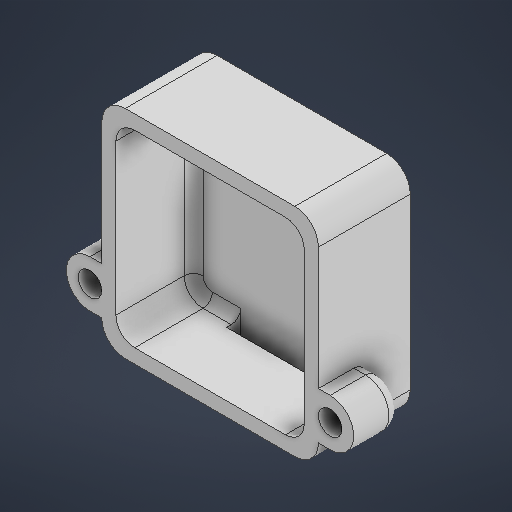
# Autodesk Inventor part: FANHOLDER
Saved by Autodesk Inventor 2025 (Build 290162010, 162A)
## iProperties
Created: 2024-04-29
Part Number: FANHOLDER
Material: Generic
Document SubType Name: Modeling
Designer: techn
Density: 1 g/cm^3
Appearance: Default
Author: techn
## iProperties of the stored document FANHOLDER_3DPrint.ipt
Created: 2024-05-28
Part Number: FANHOLDER_3DPrint
Material: Generic
Document SubType Name: Modeling
Designer: techn
Density: 1 g/cm^3
Appearance: Default
Author: techn
Autodesk Inventor part; units mm, degrees
ref_plane "YZ Plane" through (0, 0, 0) normal (1, 0, 0) x (0, 1, 0)
ref_plane "XZ Plane" through (0, 0, 0) normal (0, 1, 0) x (-1, 0, 0)
ref_plane "XY Plane" through (0, 0, 0) normal (0, 0, 1) x (1, 0, 0)
sketch "Sketch1" plane through (0, 0, 0) normal (0, 1, 0) x (-1, 0, 0)
  line L0 (0, 0) -> (-20, 0)
  line L1 (-20, 0) -> (-20, -3)
  line L2 (-20, -3) -> (0, -3)
  line L3 (0, -3) -> (0, 0)
  line L4 (3, -6) -> (-23, -6)
  line L5 (-23, -6) -> (-23, 3)
  line L6 (-23, 3) -> (3, 3)
  line L7 (3, 3) -> (3, -6)
  line L8 (-30, -6) -> (-30, 3)
  line L9 (10, 3) -> (10, -6)
  line L10 (3, -6) -> (10, -6)
  line L11 (3, 3) -> (10, 3)
  line L12 (-23, 3) -> (-30, 3)
  line L13 (-23, -6) -> (-30, -6)
  line L14 (10, -6) -> (13, -6)
  line L15 (13, -6) -> (13, 3)
  line L16 (13, 3) -> (10, 3)
  line L17 (-30, 3) -> (-33, 3)
  line L18 (-33, 3) -> (-33, -6)
  line L19 (-33, -6) -> (-30, -6)
  line L20 (0, 0) -> (10, 0)
  line L21 (0, -3) -> (10, -3)
  line L22 (-20, 0) -> (-30, 0)
  line L23 (-20, -3) -> (-30, -3)
  dimension "d0" = 20
  dimension "d1" = 3
  dimension "d2" = 3
  dimension "d6" = 40
  dimension "d7" = 3
  dimension "d8" = 3
  constraints: 48 end point, 10 point on line, 9 perpendicular, 5 parallel, 2 horizontal, 1 collinear, 3 other
  measures "d0" distance of L2.end L1.end
  measures "d1" distance of L1.end L0.end
  measures "d2" distance between parallel lines of L2 L4
  measures "d6" distance between parallel lines of L8 L9
  measures "d7" distance of L9.end L14.end
  measures "d8" distance of L8.end L17.end
extrude "Extrusion1" add sketch "Sketch1" against normal blind 3 contours L20 L7 L21 L3 | L0 L22 L5 L6 L7 L20 | L1 L23 L5 L22 | L21 L7 L4 L5 L23 L2 | L20 L9 L21 L7 | L7 L11 L9 L20 | L22 L8 L12 L5 | L5 L23 L8 L22 | L21 L9 L10 L7 | L9 L16 L15 L14 | L5 L13 L8 L23 | L8 L19 L18 L17
extrude "Extrusion2" add sketch "Sketch1" along normal blind 40 contours L0 L22 L5 L6 L7 L20 | L21 L7 L4 L5 L23 L2 | L7 L11 L9 L20 | L22 L8 L12 L5 | L21 L9 L10 L7 | L9 L16 L15 L14 | L5 L13 L8 L23 | L8 L19 L18 L17
sketch "Sketch2" plane through (0, 40, 0) normal (0, 1, 0) x (1, 0, 0)
  line L0 (33, 6) -> (-13, 6) projected
  line L1 (-13, 6) -> (-13, -3) projected
  line L2 (-13, -3) -> (33, -3) projected
  line L3 (33, -3) -> (33, 6) projected
  line L4 (-10, 3) -> (30, 3) projected
  line L5 (30, 3) -> (30, 0) projected
  line L6 (30, 0) -> (-10, 0) projected
  line L7 (-10, 0) -> (-10, 3) projected
  point P0 (0, 0)
extrude "Extrusion3" add sketch "Sketch2" along normal blind 3 contours L3 L2 L1 L0 | L4 L5 L6 L7
sketch "Sketch3" plane through (-13, -3, 3) normal (0, 0, 1) x (1, 0, 0)
  line L0 (7, 43) -> (39, 43)
  line L1 (43, 39) -> (43, 7)
  line L2 (39, 3) -> (7, 3)
  line L3 (3, 7) -> (3, 39)
  line L4 (0, 46) -> (0, 0) projected
  line L5 (46, 0) -> (0, 0) projected
  line L6 (46, 0) -> (46, 46) projected
  line L7 (0, 46) -> (46, 46) projected
  arc A0 (7, 43) -> (3, 39) centre (7, 39) ccw
  arc A1 (43, 39) -> (39, 43) centre (39, 39) ccw
  arc A2 (39, 3) -> (43, 7) centre (39, 7) ccw
  arc A3 (3, 7) -> (7, 3) centre (7, 7) ccw
  line L8 (43, 3) -> (33, 3) projected
  line L9 (43, 3) -> (39, 3)
  line L10 (43, 3) -> (43, 43) projected
  line L11 (43, 3) -> (43, 7)
  point P0 (13, 3)
  point P1 (3, 43)
  point P2 (3, 3)
  dimension "d13" = 40
  dimension "d14" = 40
  dimension "d15" = 3
  dimension "d16" = 3
  dimension "d21" = 4
  constraints: 12 end point, 10 point on circle, 10 point on line, 8 tangent, 4 centre point, 3 equal radius, 2 parallel, 1 horizontal, 1 perpendicular
  measures "d13" distance of L8.start point (3, 3)
  measures "d14" distance of L10.end L8.start
  measures "d15" distance between parallel lines of L4 L3
  measures "d16" distance between parallel lines of L7 L0
  measures "d21" radius of A0
extrude "Extrusion4" cut sketch "Sketch3" against normal blind 3 contours L0 A1 L1 A2 L2 A3 L3 A0
extrude "Extrusion6" add sketch "Sketch3" against normal blind 8 contours L10 L8 A2 | L7 L6 L5 L4
extrude "Extrusion7" add sketch "Sketch3" along normal blind 10.5 contours L10 L8 A2 | L7 L6 L5 L4
extrude "Extrusion8" cut sketch "Sketch1" against normal blind 10.5 contours L3 L2 L1 L0
fillet "Fillet1" radius 5 4 edges at (-13, 43, 3.75) (33, 43, 3.75) (-13, -3, 3.75) (33, -3, 3.75)
sketch "Sketch4" plane through (-13, -3, 13.5) normal (0, 0, 1) x (1, 0, 0)
  arc A0 (41, 0) -> (46, 5) centre (41, 5) ccw projected
  line L0 (46, 5) -> (46, 41) projected
  arc A1 (46, 41) -> (41, 46) centre (41, 41) ccw projected
  line L1 (41, 46) -> (5, 46) projected
  arc A2 (5, 46) -> (0, 41) centre (5, 41) ccw projected
  line L2 (0, 41) -> (0, 5) projected
  arc A3 (0, 5) -> (5, 0) centre (5, 5) ccw projected
  line L3 (5, 0) -> (41, 0) projected
  line L4 (7, 43) -> (39, 43) projected
  arc A4 (43, 39) -> (39, 43) centre (39, 39) ccw projected
  line L5 (43, 39) -> (43, 7) projected
  arc A5 (39, 3) -> (43, 7) centre (39, 7) ccw projected
  line L6 (39, 3) -> (7, 3) projected
  arc A6 (3, 7) -> (7, 3) centre (7, 7) ccw projected
  line L7 (3, 7) -> (3, 39) projected
  arc A7 (7, 43) -> (3, 39) centre (7, 39) ccw projected
  arc A8 (0, 5) -> (5, 0) centre (5, 5) ccw projected
  line L8 (0, 5) -> (-2.5, 5)
  line L9 (-7.5, 10) -> (-7.5, 10)
  line L10 (-2.5, 15) -> (0, 15)
  arc A9 (-2.5, 15) -> (-7.5, 10) centre (-2.5, 10) ccw
  arc A10 (-7.5, 10) -> (-2.5, 5) centre (-2.5, 10) ccw
  line L11 (46, 5) -> (48.5, 5)
  line L12 (53.5, 10) -> (53.5, 10)
  line L13 (48.5, 15) -> (46, 15)
  line L14 (46, 15) -> (46, 5)
  circle A11 centre (48.5, 10) radius 2.5
  arc A12 (53.5, 10) -> (48.5, 15) centre (48.5, 10) ccw
  arc A13 (48.5, 5) -> (53.5, 10) centre (48.5, 10) ccw
  circle A14 centre (-2.5, 10) radius 2.5
  point P0 (13, 3)
  point P1 (-7.5, 5)
  point P2 (-7.5, 15)
  point P3 (-7.5, 10)
  point P4 (53.5, 15)
  point P5 (53.5, 5)
  point P6 (53.5, 10)
  point P7 (46, 10)
  point P8 (-7.5, 10)
  point P9 (0, 10)
  dimension "d29" = 7.5
  dimension "d30" = 10
  dimension "d33" = 5
  dimension "d34" = 7.5
  dimension "d35" = 10
  dimension "d36" = 5
  dimension "d37" = 5
  dimension "d38" = 5
  dimension "d41" = 5
  constraints: 14 end point, 9 point on line, 8 point on circle, 8 tangent, 6 centre point, 3 perpendicular, 2 concentric, 2 horizontal, 2 parallel, 1 coincident, 1 midpoint, 1 vertical alignment
  measures "d29" distance of L2.end point (-7.5, 5)
  measures "d30" distance of point (-7.5, 5) point (-7.5, 15)
  measures "d33" radius of A9
  measures "d34" distance of L13.end point (53.5, 15)
  measures "d35" distance of point (53.5, 15) point (53.5, 5)
  measures "d36" diameter of A11
  measures "d37" radius of A12
  measures "d38" distance of L11.end A11.centre
  measures "d41" diameter of A14
extrude "Extrusion9" add sketch "Sketch4" against normal blind 10 contours L0 L13 A12 A13 L11 | L8 A10 A9 L10 L2
fillet "Fillet2" radius 2 3 edges at (-10, 20, -3) (10, 40, -3) (30, 20, -3)
fillet "Fillet4" radius 2.5 6 edges at (34.25, 2, 3.5) (34.25, 12, 3.5) (40.5, 7, 3.5) (-14.25, 12, 3.5) (-14.25, 2, 3.5) (-20.5, 7, 3.5)
body "Solid1"
